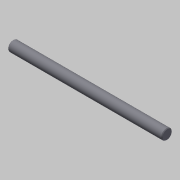
# Autodesk Inventor part: Welle 8x120mm
Saved by Autodesk Inventor 2016 (Build 200138000, 138)
## iProperties
Created: 2015-08-25
Part Number: Welle 8x120mm
Material: Steel
Document SubType Name: Modeling
Designer: 4ndreas
Density: 7.85 g/cm^3
Appearance: Steel
Mass: 47.3028 g
Surface Area: 31.0109 cm^2
Volume: 6.02584 cm^3
CustomPartVersion: 1
Author: 4ndreas
Title: Welle 8x120mm
Autodesk Inventor part; units mm, degrees
ref_plane "Startebene" through (0, 0, 0) normal (1, 0, 0) x (0, 1, 0)
ref_plane "XZ Plane" through (0, 0, 0) normal (0, 1, 0) x (-1, 0, 0)
ref_plane "XY Plane" through (0, 0, 0) normal (0, 0, 1) x (1, 0, 0)
sketch "Hauptskizze" plane through (0, 0, 0) normal (0, 0, 1) x (1, 0, 0)
  line L0 (0, 0) -> (120, 0)
  line L1 (0, 0) -> (0, 4)
  line L2 (120, 4) -> (120, 0)
  line L3 (0, 4) -> (120, 4)
  dimension "d3" = 8
  constraints: 8 end point, 2 vertical, 1 horizontal
  measures "d3" diameter of L3 L0
revolve "Umdrehung1" add sketch "Hauptskizze" angle 360 about axis through (0, 0, 0) along (1, 0, 0)
chamfer "Fase3" distance 0.5 angle 45 1 edges at (0, -4, 0) measured on face at (80, 3.987, -0.3219)
chamfer "Fase2" distance 0.5 angle 45 1 edges at (120, -4, 0) measured on face at (80.1667, 3.987, -0.3219)
